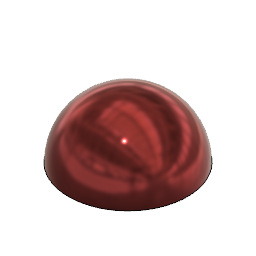
ledchaser (Autodesk Fusion 360 archive; units mm, degrees)
design "bottom"
part number: 2025-11-23-17-23-29-860
Autodesk Fusion 360 part; units mm, degrees
sphere "SpherePrimitive1" add diameter 91.567 placed x (1, 0, 0) y (0, 0, -1) z (0, 1, 0) at (0, 0, 0) makes body 1
sphere "SpherePrimitive2" cut diameter 83.567 placed x (1, 0, 0) y (0, 0, -1) z (0, 1, 0) at (0, 0, 0) bodies 1
split "Split1" by plane through (0, 0, 0) normal (0, 1, 0) bodies 1 makes body 2 at (22.6959, 5.9759, 39.3105)
move_body "Move1" bodies 2 to x (1, 0, 0) y (0, 1, 0) z (0, 0, 1) at (150, 0, 0)
delete_body "RemoveBody2" bodies 1
